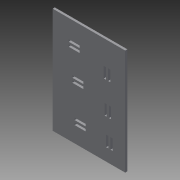
# Autodesk Inventor part: Bottom
Saved by Autodesk Inventor 2015 (Build 190159000, 159)
## iProperties
Created: 2014-09-15
Part Number: Bottom
Material: Generic
Document SubType Name: Modeling
Designer: ehagerup
Density: 1 g/cm^3
Appearance: Default
Author: ehagerup
Autodesk Inventor part; units mm, degrees
ref_plane "YZ Plane" through (0, 0, 0) normal (1, 0, 0) x (0, 1, 0)
ref_plane "XZ Plane" through (0, 0, 0) normal (0, 1, 0) x (-1, 0, 0)
ref_plane "XY Plane" through (0, 0, 0) normal (0, 0, 1) x (1, 0, 0)
sketch "Sketch1" plane through (0, 0, 0) normal (0, 1, 0) x (-1, 0, 0)
  line L0 (-7.557, 11.8403) -> (92.5214, 11.8403)
  line L1 (92.5214, 11.8403) -> (92.5214, -134.0855)
  line L2 (92.5214, -134.0855) -> (-7.557, -134.0855)
  line L3 (-7.557, -134.0855) -> (-7.557, 11.8403)
  line L4 (17.8002, -65.0745) -> (20.8002, -65.0745)
  line L5 (20.8002, -65.0745) -> (20.8002, -80.0745)
  line L6 (20.8002, -80.0745) -> (17.8002, -80.0745)
  line L7 (17.8002, -80.0745) -> (17.8002, -65.0745)
  line L8 (14.8002, -65.0745) -> (11.8002, -65.0745)
  line L9 (11.8002, -65.0745) -> (11.8002, -80.0745)
  line L10 (11.8002, -80.0745) -> (14.8002, -80.0745)
  line L11 (14.8002, -80.0745) -> (14.8002, -65.0745)
  line L12 (12.7165, -101.8292) -> (9.7165, -101.8292)
  line L13 (9.7165, -101.8292) -> (9.7165, -116.8292)
  line L14 (9.7165, -116.8292) -> (12.7165, -116.8292)
  line L15 (12.7165, -116.8292) -> (12.7165, -101.8292)
  line L16 (15.7165, -101.8292) -> (18.7165, -101.8292)
  line L17 (18.7165, -101.8292) -> (18.7165, -116.8292)
  line L18 (18.7165, -116.8292) -> (15.7165, -116.8292)
  line L19 (15.7165, -116.8292) -> (15.7165, -101.8292)
  line L20 (18.9643, -21.3009) -> (21.9643, -21.3009)
  line L21 (21.9643, -21.3009) -> (21.9643, -36.3009)
  line L22 (21.9643, -36.3009) -> (18.9643, -36.3009)
  line L23 (18.9643, -36.3009) -> (18.9643, -21.3009)
  line L24 (15.9643, -21.3009) -> (12.9643, -21.3009)
  line L25 (12.9643, -21.3009) -> (12.9643, -36.3009)
  line L26 (12.9643, -36.3009) -> (15.9643, -36.3009)
  line L27 (15.9643, -36.3009) -> (15.9643, -21.3009)
  line L28 (70.4221, -13.6009) -> (55.4221, -13.6009)
  line L29 (55.4221, -13.6009) -> (55.4221, -16.6009)
  line L30 (55.4221, -16.6009) -> (70.4221, -16.6009)
  line L31 (70.4221, -16.6009) -> (70.4221, -13.6009)
  line L32 (55.4221, -19.6009) -> (70.4221, -19.6009)
  line L33 (70.4221, -19.6009) -> (70.4221, -22.6009)
  line L34 (70.4221, -22.6009) -> (55.4221, -22.6009)
  line L35 (55.4221, -22.6009) -> (55.4221, -19.6009)
  line L36 (65.3229, -54.1341) -> (50.3229, -54.1341)
  line L37 (50.3229, -54.1341) -> (50.3229, -57.1341)
  line L38 (50.3229, -57.1341) -> (65.3229, -57.1341)
  line L39 (65.3229, -57.1341) -> (65.3229, -54.1341)
  line L40 (50.3229, -60.1341) -> (65.3229, -60.1341)
  line L41 (65.3229, -60.1341) -> (65.3229, -63.1341)
  line L42 (65.3229, -63.1341) -> (50.3229, -63.1341)
  line L43 (50.3229, -63.1341) -> (50.3229, -60.1341)
  line L44 (47.1773, -103.1635) -> (62.1773, -103.1635)
  line L45 (62.1773, -103.1635) -> (62.1773, -106.1635)
  line L46 (62.1773, -106.1635) -> (47.1773, -106.1635)
  line L47 (47.1773, -106.1635) -> (47.1773, -103.1635)
  line L48 (62.1773, -109.1635) -> (47.1773, -109.1635)
  line L49 (47.1773, -109.1635) -> (47.1773, -112.1635)
  line L50 (47.1773, -112.1635) -> (62.1773, -112.1635)
  line L51 (62.1773, -112.1635) -> (62.1773, -109.1635)
  point P0 (0, 0)
  constraints: 104 end point, 26 parallel, 13 horizontal, 13 perpendicular
extrude "Extrusion1" add sketch "Sketch1" along normal blind 3
body "Solid1"
